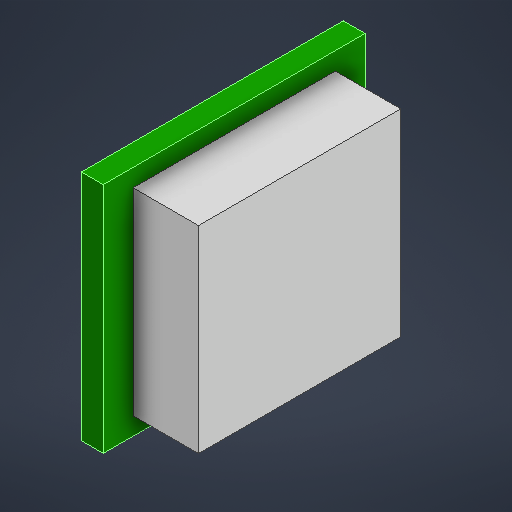
# Autodesk Inventor part: P_driver
Saved by Autodesk Inventor 2026.2 (Build 302298000, 298)
## iProperties
Created: 2026-02-21
Part Number: P_driver
Material: Generisch
Document SubType Name: Modeling
Designer: FAL
Density: 1 g/cm^3
Appearance: Vorgabe
Author: FAL
Autodesk Inventor part; units mm, degrees
ref_plane "YZ Plane" through (0, 0, 0) normal (1, 0, 0) x (0, 1, 0)
ref_plane "XZ Plane" through (0, 0, 0) normal (0, 1, 0) x (-1, 0, 0)
ref_plane "XY Plane" through (0, 0, 0) normal (0, 0, 1) x (1, 0, 0)
sketch "Skizze1" plane through (0, 0, 0) normal (1, 0, 0) x (0, 1, 0)
  line L0 (9, -8) -> (-9, -8)
  line L1 (-9, -8) -> (-9, 8)
  line L2 (-9, 8) -> (9, 8)
  line L3 (9, 8) -> (9, -8)
  line L4 (9, -8) -> (-9, 8) construction
  line L5 (-9, -8) -> (9, 8) construction
  point P0 (0, 0)
  dimension "d0" = 16
  dimension "d1" = 18
  constraints: 12 end point, 2 midpoint, 2 parallel, 1 horizontal, 1 perpendicular
  measures "d0" distance of L2.end L0.start
  measures "d1" distance between parallel lines of L1 L3
extrude "Extrusion1" add sketch "Skizze1" along normal blind 1.5
sketch "Skizze2" plane through (1.5, 0, 0) normal (1, 0, 0) x (0, 0, -1)
  line L0 (6.7859, 6.9513) -> (-6.7859, 6.9513)
  line L1 (-6.7859, 6.9513) -> (-6.7859, -6.9513)
  line L2 (-6.7859, -6.9513) -> (6.7859, -6.9513)
  line L3 (6.7859, -6.9513) -> (6.7859, 6.9513)
  line L4 (6.7859, 6.9513) -> (-6.7859, -6.9513) construction
  line L5 (-6.7859, 6.9513) -> (6.7859, -6.9513) construction
  point P0 (0, 0)
  constraints: 12 end point, 2 midpoint, 2 parallel, 1 horizontal, 1 perpendicular
extrude "Extrusion2" add sketch "Skizze2" along normal blind 4.5 separate body
